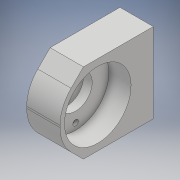
# Autodesk Inventor part: Porte_encodeur
Saved by Autodesk Inventor 2018 (Build 220112000, 112)
## iProperties
Created: 2019-11-11
Part Number: Porte_encodeur
Material: Generic
Document SubType Name: Modeling
Designer: hugo
Density: 1 g/cm^3
Appearance: Default
Author: hugo
Autodesk Inventor part; units mm, degrees
ref_plane "YZ Plane" through (0, 0, 0) normal (1, 0, 0) x (0, 1, 0)
ref_plane "XZ Plane" through (0, 0, 0) normal (0, 1, 0) x (-1, 0, 0)
ref_plane "XY Plane" through (0, 0, 0) normal (0, 0, 1) x (1, 0, 0)
sketch "Sketch1" plane through (0, 0, 0) normal (1, 0, 0) x (0, 1, 0)
  circle A0 centre (17, 0) radius 15 construction
  line L0 (42, 0) -> (42, 18)
  line L1 (42, 18) -> (10.539, 18)
  line L2 (10.539, 18) -> (0, 7.461)
  line L3 (0, 7.461) -> (0, 0)
  line L4 (42, 0) -> (0, 0) construction
  line L5 (42, 0) -> (42, -18)
  line L6 (42, -18) -> (10.539, -18)
  line L7 (10.539, -18) -> (0, -7.461)
  line L8 (0, -7.461) -> (0, 0)
  line L9 (0, 15.5075) -> (0, -16.6542) construction
  dimension "d0" = 30
  dimension "d1" = 17
  dimension "d2" = 25
  dimension "d3" = 18
  dimension "d5" = 135
  constraints: 20 end point, 3 symmetric about line, 2 horizontal, 2 point on line, 2 vertical, 1 centre point
  measures "d0" diameter of A0
  measures "d1" distance of L3.end A0.centre
  measures "d2" distance of A0.centre L0.start
  measures "d3" distance of L0.start L0.end
  measures "d5" angle of L2 L1
extrude "Extrusion1" add sketch "Sketch1" along normal blind 15
sketch "Sketch2" plane through (15, 0, 0) normal (1, 0, 0) x (0, 0, -1)
  circle A0 centre (0, 17) radius 15
  point P0 (0, 0)
  dimension "d8" = 30
  dimension "d9" = 17
  constraints: 1 centre point
  measures "d8" diameter of A0
  measures "d9" distance of point (0, 0) A0.centre
extrude "Extrusion2" cut sketch "Sketch2" against normal blind 10
sketch "Sketch3" plane through (5, 17, 0) normal (1, 0, 0) x (0, 0, -1)
  circle A0 centre (0, 0) radius 7.5
  point P0 (0, -17)
  dimension "d12" = 15
  constraints: 1 centre point
  measures "d12" diameter of A0
extrude "Extrusion3" cut sketch "Sketch3" against normal blind 4
sketch "Sketch4" plane through (1, 17, 0) normal (1, 0, 0) x (0, 0, -1)
  circle A0 centre (0, 0) radius 7.5 projected
  circle A1 centre (0, 0) radius 2.25
  point P0 (0, -17)
  dimension "d15" = 4.5
  constraints: 1 centre point, 1 coincident
  measures "d15" diameter of A1
extrude "Extrusion4" cut sketch "Sketch4" against normal up to next contours A1
sketch "Sketch5" plane through (0, 0, 0) normal (-1, 0, 0) x (0, 0, 1)
  circle A0 centre (0, 17) radius 2.25 projected
  circle A1 centre (0, 17) radius 12 construction
  point P0 (0, 0)
  point P1 (-12, 17)
  point P2 (12, 17)
  dimension "d18" = 24
  constraints: 2 point on circle, 1 centre point, 1 coincident
  measures "d18" diameter of A1
hole "Hole1" at (0, 17, -12) at (0, 17, 12) direction (1, 0, 0) diameter 2.459 end through all counterbore diameter 6 counterbore depth 3.5
sketch "Sketch6" plane through (0, 42, 18) normal (0, 1, 0) x (1, 0, 0)
  line L0 (0, 18) -> (15, 18) construction
  line L1 (15, 10.539) -> (15, 25.461) construction
  line L2 (15, 36) -> (15, 0) construction
  point P0 (9, 5.5)
  point P1 (9, 30.5)
  dimension "d26" = 12.5
  dimension "d27" = 6
  constraints: 2 end point, 1 midpoint, 1 symmetric about line
  measures "d26" distance from line of L0 point (9, 5.5)
  measures "d27" distance from line of L2 point (9, 5.5)
hole "Hole2" at (9, 42, 12.5) at (9, 42, -12.5) direction (0, -1, 0) diameter 4.917 depth 5 tip angle 118 thread size "M6x1" class "6H" standard "ISO Metric profile"
fillet "Fillet1" radius 17 2 edges at (7.5, 0, -7.461) (7.5, 0, 7.461)
body "Solid1"
